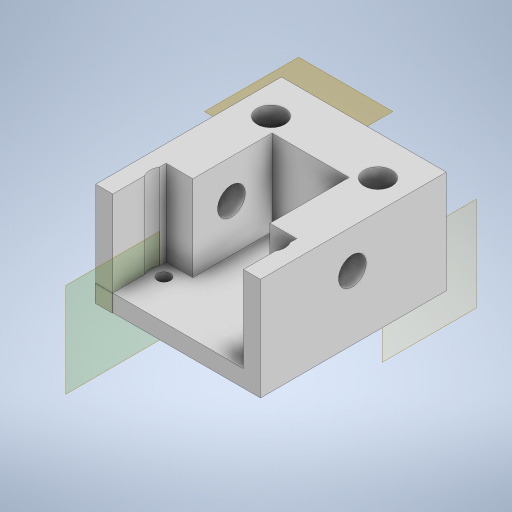
# Autodesk Inventor part: linrail_mov_holder_ax
Saved by Autodesk Inventor 2024 (Build 280153000, 153)
## iProperties
Created: 2025-12-26
Part Number: linrail_mov_holder_ax
Material: Generic
Document SubType Name: Modeling
Designer: schar
Density: 1 g/cm^3
Appearance: Default
Author: schar
Autodesk Inventor part; units mm, degrees
ref_plane "YZ Plane" through (0, 0, 0) normal (1, 0, 0) x (0, 1, 0)
ref_plane "XZ Plane" through (0, 0, 0) normal (0, 1, 0) x (-1, 0, 0)
ref_plane "XY Plane" through (0, 0, 0) normal (0, 0, 1) x (1, 0, 0)
ref_plane "Work Plane1" through (-15.25, 11.25, -51.1) normal (0, 1, 0) x (1, 0, 0)
sketch "Sketch1" plane through (-15.25, 11.25, -51.1) normal (0, 1, 0) x (1, 0, 0)
  line L0 (0, 0) -> (-1, 0) projected
  line L1 (30.5, 0) -> (30.5, -43.4) projected
  line L2 (0, 0) -> (30.5, 0)
  line L3 (30.5, 0) -> (30.5, -43.4)
  line L4 (30.5, -43.4) -> (0, -43.4)
  line L5 (0, -43.4) -> (0, 0)
  circle A0 centre (2.75, -9.2) radius 1.5 projected
  circle A1 centre (2.75, -9.2) radius 1.5
  circle A2 centre (2.75, -34.2) radius 1.5 projected
  circle A3 centre (2.75, -34.2) radius 1.5
  circle A4 centre (27.75, -34.2) radius 1.5 projected
  circle A5 centre (27.75, -34.2) radius 1.5
  circle A6 centre (27.75, -9.2) radius 1.5 projected
  circle A7 centre (27.75, -9.2) radius 1.5
  point P0 (15.25, -51.1)
  constraints: 8 end point, 4 centre point, 4 coincident, 2 parallel, 1 horizontal, 1 perpendicular
extrude "Extrusion1" add sketch "Sketch1" along normal blind 4
ref_plane "Work Plane2" through (-15.25, 11.25, -7.7) normal (-1, 0, 0) x (0, 0, 1)
sketch "Sketch2" plane through (-15.25, 11.25, -7.7) normal (-1, 0, 0) x (0, 0, 1)
  line L0 (-43.4, 0) -> (-43.4, 4) projected
  line L1 (-43.4, 0) -> (0.1445, 0)
  line L2 (0.1445, 0) -> (0.1445, 4)
  line L3 (0.1445, 4) -> (-43.4, 4)
  line L4 (-43.4, 4) -> (-43.4, 0)
  point P0 (7.7, -11.25)
  constraints: 8 end point, 2 parallel, 1 horizontal, 1 perpendicular
extrude "Extrusion2" add sketch "Sketch2" along normal blind 4
ref_plane "Work Plane3" through (15.25, 11.25, -51.1) normal (1, 0, 0) x (0, 0, -1)
sketch "Sketch3" plane through (15.25, 11.25, -51.1) normal (1, 0, 0) x (0, 0, -1)
  line L0 (0, 0) -> (0, 4) projected
  line L1 (0, 4) -> (-43.4, 4)
  line L2 (-43.4, 4) -> (-43.4, 0.0024)
  line L3 (-43.4, 0.0024) -> (0, 0.0024)
  line L4 (0, 0.0024) -> (0, 4)
  point P0 (-51.1, -11.25)
  constraints: 8 end point, 2 parallel, 1 horizontal, 1 perpendicular
extrude "Extrusion3" add sketch "Sketch3" along normal blind 4
ref_plane "Work Plane6" through (-15.25, 15.25, -51.1) normal (0, 1, 0) x (1, 0, 0)
sketch "Sketch4" plane through (-15.25, 15.25, -51.1) normal (0, 1, 0) x (1, 0, 0)
  line L0 (-0.75, -43.4) -> (0.25, -43.4) projected
  line L1 (-0.0048, -43.4) -> (-4, -43.4)
  line L2 (-4, -43.4) -> (-4, 0)
  line L3 (-4, 0) -> (-0.0048, 0)
  line L4 (-0.0048, 0) -> (-0.0048, -43.4)
  point P0 (15.25, -51.1)
  constraints: 8 end point, 2 parallel, 1 horizontal, 1 perpendicular, 1 point on line
extrude "Extrusion4" add sketch "Sketch4" along normal blind 15
ref_plane "Work Plane5" through (-15.25, 15.25, -51.1) normal (0, 1, 0) x (1, 0, 0)
sketch "Sketch5" plane through (-15.25, 15.25, -51.1) normal (0, 1, 0) x (1, 0, 0)
  line L0 (30.5, 0) -> (34.5, 0) projected
  line L1 (30.5, -43.4) -> (30.5, 0) projected
  line L2 (34.5, 0) -> (30.5, 0)
  line L3 (30.5, 0) -> (30.5, -43.4)
  line L4 (30.5, -43.4) -> (34.5, -43.4)
  line L5 (34.5, -43.4) -> (34.5, 0)
  point P0 (15.25, -51.1)
  constraints: 8 end point, 2 parallel, 1 horizontal, 1 perpendicular
extrude "Extrusion5" add sketch "Sketch5" along normal blind 15
ref_plane "Work Plane4" through (-15.25, 15.25, -51.1) normal (0, 1, 0) x (1, 0, 0)
sketch "Sketch6" plane through (-15.25, 15.25, -51.1) normal (0, 1, 0) x (1, 0, 0)
  circle A0 centre (2.75, -34.2) radius 2 projected
  circle A1 centre (2.75, -34.2) radius 3.25
  circle A2 centre (27.75, -34.2) radius 1.5 projected
  circle A3 centre (27.75, -34.2) radius 3.25
  circle A4 centre (27.75, -9.2) radius 1.5 projected
  circle A5 centre (27.75, -9.2) radius 3.25
  circle A6 centre (2.75, -9.2) radius 1.5 projected
  circle A7 centre (2.75, -9.2) radius 3.25
  line L0 (15.25, -21.7) -> (24.25, -21.7)
  line L1 (15.25, -21.7) -> (6.25, -21.7)
  line L2 (30.5, 0) -> (30.5, -43.4) projected
  line L3 (24.25, -21.7) -> (30.5, -21.7)
  line L4 (30.5, -21.7) -> (30.5, -12.45)
  line L5 (30.5, -12.45) -> (24.25, -12.45)
  line L6 (24.25, -12.45) -> (24.25, -21.7)
  line L7 (24.25, -21.7) -> (30.5, -21.7)
  line L8 (30.5, -21.7) -> (30.5, -30.95)
  line L9 (30.5, -30.95) -> (24.25, -30.95)
  line L10 (24.25, -30.95) -> (24.25, -21.7)
  line L11 (-0.0048, 0) -> (-0.0048, -43.4) projected
  line L12 (6.25, -21.7) -> (-0.0048, -21.7)
  line L13 (-0.0048, -21.7) -> (-0.0048, -30.95)
  line L14 (-0.0048, -30.95) -> (6.25, -30.95)
  line L15 (6.25, -30.95) -> (6.25, -21.7)
  line L16 (6.25, -21.7) -> (-0.0048, -21.7)
  line L17 (-0.0048, -21.7) -> (-0.0048, -12.45)
  line L18 (-0.0048, -12.45) -> (6.25, -12.45)
  line L19 (6.25, -12.45) -> (6.25, -21.7)
  point P0 (15.25, -51.1)
  dimension "d11" = 6.5
  dimension "d12" = 6.5
  dimension "d13" = 6.5
  dimension "d14" = 6.5
  dimension "d15" = 9
  dimension "d16" = 9
  constraints: 36 end point, 8 parallel, 6 horizontal, 6 point on line, 4 centre point, 4 coincident, 4 perpendicular
  measures "d11" diameter of A1
  measures "d12" diameter of A3
  measures "d13" diameter of A5
  measures "d14" diameter of A7
  measures "d15" distance of L0.start L0.end
  measures "d16" distance of L0.start L1.end
extrude "Extrusion6" add sketch "Sketch6" along normal blind 15 contours L14 L11 L12 L15 | L11 L18 L19 L12 | L9 L10 L3 L2 | L3 L6 L5 L2
ref_plane "Work Plane8" through (-15.25, 30.25, -51.1) normal (0, 1, 0) x (1, 0, 0)
sketch "Sketch7" plane through (-15.25, 30.25, -51.1) normal (0, 1, 0) x (1, 0, 0)
  line L0 (0, -43.4) -> (0, -43.5445) projected
  line L1 (-4, -43.4) -> (-0.0048, -43.4) projected
  line L2 (0, -43.4) -> (-4, -43.4)
  line L3 (-0.0048, 0) -> (-4, 0) projected
  line L4 (-4, -43.4) -> (-4, 0)
  line L5 (-4, 0) -> (-0.0048, 0)
  line L6 (-0.0048, -12.45) -> (-0.0048, 0) projected
  line L7 (-0.0048, 0) -> (-0.0048, -12.45)
  line L8 (6.25, -30.95) -> (6.25, -12.45) projected
  line L9 (-0.0048, -12.45) -> (6.25, -12.45)
  line L10 (6.25, -12.45) -> (6.25, -30.95)
  line L11 (-0.0048, -30.95) -> (-0.0048, -43.4) projected
  line L12 (6.25, -30.95) -> (-0.0048, -30.95)
  line L13 (-0.0048, -30.95) -> (-0.0048, -43.4)
  line L14 (24.25, -12.45) -> (24.25, -30.95) projected
  line L15 (24.25, -30.95) -> (24.25, -12.45)
  line L16 (30.5, -12.45) -> (24.25, -12.45) projected
  line L17 (24.25, -12.45) -> (30.5, -12.45)
  line L18 (30.5, -12.45) -> (30.5, 0)
  line L19 (30.5, 0) -> (34.4541, 0)
  line L20 (34.4541, 0) -> (34.4541, -43.4)
  line L21 (34.4541, -43.4) -> (30.5, -43.4)
  line L22 (30.5, -43.4) -> (30.5, -30.95)
  line L23 (30.5, -30.95) -> (24.25, -30.95)
  point P0 (15.25, -51.1)
  constraints: 32 end point, 11 perpendicular, 2 point on line, 2 vertical, 1 collinear, 1 horizontal
extrude "Extrusion7" add sketch "Sketch7" along normal blind 5
ref_plane "Work Plane7" through (-15.25, 30.25, -51.1) normal (0, 1, 0) x (1, 0, 0)
sketch "Sketch8" plane through (-15.25, 30.25, -51.1) normal (0, 1, 0) x (1, 0, 0)
  line L0 (30.5, -43.4) -> (34.5, -43.4) projected
  line L1 (34.4541, 0) -> (34.4541, -43.4) projected
  line L2 (34.5, -43.4) -> (34.4541, -43.4)
  line L3 (34.4541, -43.4) -> (34.4541, 0)
  line L4 (34.4541, 0) -> (34.5, 0)
  line L5 (34.5, 0) -> (34.5, -43.4)
  point P0 (15.25, -51.1)
  constraints: 8 end point, 2 parallel, 1 horizontal, 1 perpendicular
extrude "Extrusion8" add sketch "Sketch8" along normal blind 5
ref_plane "Work Plane9" through (-15.2548, 15.25, -38.65) normal (1, 0, 0) x (0, 0, -1)
sketch "Sketch9" plane through (-15.2548, 15.25, -38.65) normal (1, 0, 0) x (0, 0, -1)
  line L0 (0, 0) -> (0, 20) projected
  line L1 (12.45, 20) -> (0, 20) projected
  line L2 (0, 0) -> (12.45, 0)
  line L3 (12.45, 0) -> (12.45, 20)
  line L4 (12.45, 20) -> (0, 20)
  line L5 (0, 20) -> (0, 0)
  point P0 (-38.65, -15.25)
  constraints: 8 end point, 2 parallel, 1 horizontal, 1 perpendicular
extrude "Extrusion9" add sketch "Sketch9" along normal up to surface (30.5048 mm away)
sketch "Sketch10" plane through (-15.25, 11.25, -51.1) normal (0, -1, 0) x (1, 0, 0)
  circle A0 centre (27.75, 9.2) radius 1.5 projected
  circle A1 centre (27.75, 9.2) radius 1.5
  circle A2 centre (2.75, 9.2) radius 1.5 projected
  circle A3 centre (2.75, 9.2) radius 1.5
  point P0 (15.25, 51.1)
  constraints: 2 centre point, 2 coincident
extrude "Extrusion10" cut sketch "Sketch10" against normal through all
sketch "Sketch11" plane through (-15.25, 35.25, -51.1) normal (0, 1, 0) x (1, 0, 0)
  circle A0 centre (2.75, -9.2) radius 1.5 projected
  circle A1 centre (2.75, -9.2) radius 3.25
  circle A2 centre (27.75, -9.2) radius 1.5 projected
  circle A3 centre (27.75, -9.2) radius 3.25
  circle A4 centre (2.75, -34.2) radius 1.5 projected
  circle A5 centre (2.75, -34.2) radius 3.25
  circle A6 centre (27.75, -34.2) radius 1.5 projected
  circle A7 centre (27.75, -34.2) radius 3.25
  point P0 (15.25, -51.1)
  dimension "d27" = 6.5
  dimension "d28" = 6.5
  dimension "d29" = 6.5
  dimension "d30" = 6.5
  constraints: 4 centre point, 4 coincident
  measures "d27" diameter of A1
  measures "d28" diameter of A3
  measures "d29" diameter of A5
  measures "d30" diameter of A7
extrude "Extrusion11" cut sketch "Sketch11" against normal up to surface (20 mm away) contours A0 | A1 | A2 | A3 | A4 | A5 | A6 | A7
sketch "Sketch12" plane through (9, 15.25, -20.15) normal (-1, 0, 0) x (0, 0, 1)
  line L0 (0, 20) -> (0, 0) projected
  line L1 (0, 20) -> (0, 11)
  line L2 (0, 11) -> (-9, 11)
  circle A0 centre (-9, 11) radius 3.25
  point P0 (20.15, -15.25)
  dimension "d33" = 9
  dimension "d34" = 9
  dimension "d35" = 6.5
  constraints: 4 end point, 1 centre point, 1 coincident, 1 perpendicular, 1 point on line
  measures "d33" distance of L0.start L1.end
  measures "d34" distance of L1.end L2.end
  measures "d35" diameter of A0
extrude "Extrusion12" cut sketch "Sketch12" along normal mid plane 70
body "Solid2"
